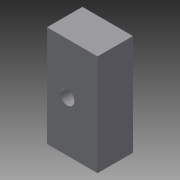
# Autodesk Inventor part: NailBitHold
Saved by Autodesk Inventor 2015 (Build 190159000, 159)
## iProperties
Created: 2016-03-24
Part Number: NailBitHold
Material: Generic
Document SubType Name: Modeling
Designer: Hatch
Density: 1 g/cm^3
Appearance: Default
Author: Hatch
Autodesk Inventor part; units mm, degrees
ref_plane "YZ Plane" through (0, 0, 0) normal (1, 0, 0) x (0, 1, 0)
ref_plane "XZ Plane" through (0, 0, 0) normal (0, 1, 0) x (-1, 0, 0)
ref_plane "XY Plane" through (0, 0, 0) normal (0, 0, 1) x (1, 0, 0)
sketch "Sketch1" plane through (0, 0, 0) normal (0, 1, 0) x (-1, 0, 0)
  line L0 (-7.25, 7.25) -> (7.25, 7.25)
  line L1 (7.25, 7.25) -> (7.25, -7.25)
  line L2 (7.25, -7.25) -> (-7.25, -7.25)
  line L3 (-7.25, -7.25) -> (-7.25, 7.25)
  line L4 (-7.25, 7.25) -> (7.25, -7.25) construction
  line L5 (7.25, 7.25) -> (-7.25, -7.25) construction
  point P0 (0, 0)
  dimension "d0" = 14.5
  dimension "d1" = 14.5
  constraints: 12 end point, 2 midpoint, 2 parallel, 1 horizontal, 1 perpendicular
  measures "d0" distance of L1.end L2.end
  measures "d1" distance of L0.end L1.end
extrude "Extrusion1" add sketch "Sketch1" along normal blind 76.2
sketch "Sketch2" plane through (0, 76.2, 0) normal (0, 1, 0) x (1, 0, 0)
  line L0 (10, -10) -> (-10, -10)
  line L1 (-10, -10) -> (-10, 10)
  line L2 (-10, 10) -> (10, 10)
  line L3 (10, 10) -> (10, -10)
  line L4 (10, -10) -> (-10, 10) construction
  line L5 (-10, -10) -> (10, 10) construction
  point P0 (0, 0)
  dimension "d4" = 20
  dimension "d5" = 20
  constraints: 12 end point, 2 midpoint, 2 parallel, 1 horizontal, 1 perpendicular
  measures "d4" distance of L1.end L2.end
  measures "d5" distance of L0.end L1.end
extrude "Extrusion2" add sketch "Sketch2" along normal blind 5
sketch "Sketch3" plane through (0, 81.2, 0) normal (0, 1, 0) x (1, 0, 0)
  line L0 (7.5, -7.5) -> (-7.5, -7.5)
  line L1 (-7.5, -7.5) -> (-7.5, 7.5)
  line L2 (-7.5, 7.5) -> (7.5, 7.5)
  line L3 (7.5, 7.5) -> (7.5, -7.5)
  line L4 (7.5, -7.5) -> (-7.5, 7.5) construction
  line L5 (-7.5, -7.5) -> (7.5, 7.5) construction
  line L6 (10, -10) -> (-10, -10)
  line L7 (-10, -10) -> (-10, 10)
  line L8 (-10, 10) -> (10, 10)
  line L9 (10, 10) -> (10, -10)
  line L10 (10, -10) -> (-10, 10) construction
  line L11 (-10, -10) -> (10, 10) construction
  point P0 (0, 0)
  dimension "d8" = 15
  dimension "d9" = 15
  constraints: 24 end point, 4 midpoint, 4 parallel, 2 horizontal, 2 perpendicular
  measures "d8" distance of L1.end L2.end
  measures "d9" distance of L0.end L1.end
extrude "Extrusion3" add sketch "Sketch3" along normal blind 76.2
sketch "Sketch4" plane through (10, 76.2, 10) normal (1, 0, 0) x (0, 0, -1)
  line L0 (20, 0) -> (20, 81.2) projected
  line L1 (15, 81.2) -> (15, 0)
  line L2 (0, 0) -> (20, 0) projected
  line L3 (15, 81.2) -> (13, 81.2)
  line L4 (17.5, 81.2) -> (2.5, 81.2) projected
  line L5 (13, 81.2) -> (13, 0)
  line L6 (13, 0) -> (15, 0)
  line L7 (20, 81.2) -> (0, 81.2) projected
  point P0 (10, -76.2)
  dimension "d12" = 2
  constraints: 8 end point, 3 point on line, 1 parallel, 1 perpendicular, 1 vertical
  measures "d12" distance of L1.start L3.end
extrude "Extrusion4" add sketch "Sketch4" along normal blind 10 contours L2 L5 L3 L1
sketch "Sketch5" plane through (10, 76.2, -3) normal (0, 0, 1) x (1, 0, 0)
  line L0 (0, 81.2) -> (10, 81.2) projected
  line L1 (10, 81.2) -> (8, 81.2)
  line L2 (8, 81.2) -> (8, 0)
  line L3 (8, 0) -> (10, 0)
  line L4 (10, 0) -> (10, 81.2)
  point P0 (-10, -76.2)
  dimension "d15" = 2
  constraints: 8 end point, 2 parallel, 1 perpendicular, 1 point on line
  measures "d15" distance of L0.end L1.end
extrude "Extrusion5" add sketch "Sketch5" along normal blind 8
sketch "Sketch6" plane through (20, 76.2, 10) normal (1, 0, 0) x (0, 0, -1)
  line L0 (5, 81.2) -> (3, 81.2)
  line L1 (3, 81.2) -> (3, 0)
  line L2 (3, 0) -> (5, 0)
  line L3 (5, 0) -> (5, 81.2)
  point P0 (10, -76.2)
  dimension "d18" = 2
  constraints: 8 end point, 2 parallel, 1 horizontal, 1 perpendicular
  measures "d18" distance of L0.start L0.end
extrude "Extrusion6" add sketch "Sketch6" against normal blind 4
sketch "Sketch7" plane through (0, 76.2, 0) normal (0, -1, 0) x (1, 0, 0)
  line L0 (10, -5) -> (20, -5)
  line L1 (20, -5) -> (20, 7)
  line L2 (20, 7) -> (10, 7)
  line L3 (10, 7) -> (10, -5)
  point P0 (0, 0)
  constraints: 8 end point, 2 parallel, 1 horizontal, 1 perpendicular
extrude "Extrusion7" cut sketch "Sketch7" against normal through all
sketch "Sketch8" plane through (7.25, 0, -7.25) normal (0, 0, -1) x (-1, 0, 0)
  line L0 (0, 0) -> (0, 76.2)
  line L1 (0, 0) -> (0, 76.2) projected
  line L2 (0, 38.1) -> (14.5, 38.1)
  line L3 (14.5, 38.1) -> (14.5, 0)
  line L4 (14.5, 0) -> (0, 0)
  line L5 (0, 0) -> (0, 38.1)
  point P0 (7.25, 0)
  constraints: 10 end point, 3 equal length, 1 horizontal, 1 midpoint, 1 perpendicular
extrude "Extrusion8" cut sketch "Sketch8" against normal through all
sketch "Sketch9" plane through (10, 76.2, -10) normal (0, 0, -1) x (-1, 0, 0)
  line L0 (0, 0) -> (0, 20)
  line L1 (0, 0) -> (0, 81.2) projected
  line L2 (0, 20) -> (20, 20)
  line L3 (20, 20) -> (20, 81.2)
  line L4 (20, 81.2) -> (0, 81.2)
  line L5 (0, 81.2) -> (0, 20)
  point P0 (10, -76.2)
  dimension "d25" = 20
  constraints: 10 end point, 2 parallel, 1 horizontal, 1 perpendicular, 1 point on line
  measures "d25" distance of L0.start L0.end
extrude "Extrusion9" cut sketch "Sketch9" against normal through all
sketch "Sketch10" plane through (-10, 96.2, -10) normal (0, 1, 0) x (1, 0, 0)
  line L0 (17.5, -2.5) -> (2.5, -2.5)
  line L1 (2.5, -2.5) -> (2.5, -17.5)
  line L2 (2.5, -17.5) -> (17.5, -17.5)
  line L3 (17.5, -17.5) -> (17.5, -2.5)
  point P0 (10, -10)
  constraints: 8 end point, 2 parallel, 1 horizontal, 1 perpendicular
extrude "Extrusion10" add sketch "Sketch10" against normal blind 15
sketch "Sketch12" plane through (10, 76.2, 10) normal (1, 0, 0) x (0, 0, -1)
  line L0 (20, 20) -> (9, 20)
  line L1 (20, 20) -> (0, 20) projected
  line L2 (2.75, 0) -> (17.25, 0) projected
  line L3 (20, 20) -> (13, 20)
  line L4 (13, 20) -> (13, 0)
  line L5 (13, 0) -> (20, 0)
  line L6 (20, 0) -> (20, 20)
  point P0 (10, -76.2)
  dimension "d30" = 11
  dimension "d31" = 7
  constraints: 10 end point, 2 parallel, 2 point on line, 1 horizontal, 1 perpendicular
  measures "d30" distance of L0.start L0.end
  measures "d31" distance of L5.end L4.end
extrude "Extrusion11" add sketch "Sketch12" along normal blind 10
sketch "Sketch13" plane through (-10, 76.2, -10) normal (0, 0, -1) x (-1, 0, 0)
  line L0 (-17.25, 0) -> (-17.25, 20)
  line L1 (0, 20) -> (-30, 20) projected
  line L2 (-17.25, -38.1) -> (-17.25, 0) projected
  line L3 (-20, 0) -> (-20, 20)
  line L4 (-20, 0) -> (-20, 20) projected
  line L5 (-20, 10) -> (-24, 10)
  circle A0 centre (-24, 10) radius 1.4
  point P0 (-10, -76.2)
  dimension "d34" = 4
  dimension "d35" = 2.8
  constraints: 6 end point, 2 collinear, 1 centre point, 1 coincident, 1 horizontal, 1 midpoint, 1 point on line
  measures "d34" distance of L5.start L5.end
  measures "d35" diameter of A0
extrude "Extrusion12" cut sketch "Sketch13" against normal through all
sketch "Sketch14" plane through (-10, 76.2, 10) normal (0, 0, 1) x (1, 0, 0)
  line L0 (20, 20) -> (-2.0792, 20)
  line L1 (-2.0792, 20) -> (-2.0792, -41.5278)
  line L2 (-2.0792, -41.5278) -> (20, -41.5278)
  line L3 (20, -41.5278) -> (20, 20)
  point P0 (10, -76.2)
  constraints: 8 end point, 2 parallel, 1 horizontal, 1 perpendicular
extrude "Extrusion13" cut sketch "Sketch14" against normal through all
body "Solid1"
